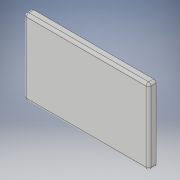
# Autodesk Inventor part: 時鐘底座
Saved by Autodesk Inventor 2019 (Build 230136000, 136)
## iProperties
Created: 2019-01-20
Part Number: 時鐘底座
Material: 一般
Document SubType Name: Modeling
Designer: j13tw
Density: 1 g/cm^3
Appearance: 預設
Author: j13tw
Autodesk Inventor part; units mm, degrees
ref_plane "YZ Plane" through (0, 0, 0) normal (1, 0, 0) x (0, 1, 0)
ref_plane "XZ Plane" through (0, 0, 0) normal (0, 1, 0) x (-1, 0, 0)
ref_plane "XY Plane" through (0, 0, 0) normal (0, 0, 1) x (1, 0, 0)
sketch "草圖1" plane through (0, 0, 0) normal (0, 0, 1) x (1, 0, 0)
  line L0 (0, 0) -> (50, 0)
  line L1 (50, 0) -> (50, 30.17)
  line L2 (50, 30.17) -> (0, 30.17)
  line L3 (0, 30.17) -> (0, 0)
  dimension "d0" = 30.17
  dimension "d1" = 50
  constraints: 8 end point, 2 parallel, 1 horizontal, 1 perpendicular
  measures "d0" distance of L0.end L1.end
  measures "d1" distance of L1.end L2.end
extrude "擠出1" add sketch "草圖1" along normal blind 3
fillet "圓角1" radius 1 4 edges at (25, 0, 3) (25, 30.17, 3) (50, 15.085, 3) (0, 15.085, 3)
fillet "圓角2" radius 1 2 edges at (0, 0, 1) (0.2929, 0.2929, 2.7071)
fillet "圓角3" radius 1 2 edges at (0.2929, 29.8771, 2.7071) (0, 30.17, 1)
fillet "圓角4" radius 1 4 edges at (49.7071, 0.2929, 2.7071) (50, 0, 1) (49.7071, 29.8771, 2.7071) (50, 30.17, 1)
